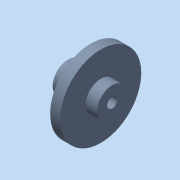
# Autodesk Inventor part: Kupplung
Saved by Autodesk Inventor 2015 (Build 190159000, 159)
## iProperties
Created: 2017-11-12
Part Number: Kupplung
Material: Generisch
Document SubType Name: Modeling
Designer: Christoph Soppa
Density: 1 g/cm^3
Appearance: Stahlblau - hell
Author: Christoph Soppa
Autodesk Inventor part; units mm, degrees
ref_plane "YZ Plane" through (0, 0, 0) normal (1, 0, 0) x (0, 1, 0)
ref_plane "XZ Plane" through (0, 0, 0) normal (0, 1, 0) x (-1, 0, 0)
ref_plane "XY Plane" through (0, 0, 0) normal (0, 0, 1) x (1, 0, 0)
sketch "Skizze1" plane through (0, 0, 0) normal (0, 0, 1) x (1, 0, 0)
  line L0 (0, 0) -> (16.2131, 0)
  line L1 (0, 2) -> (17.5, 2)
  line L2 (17.5, 2) -> (17.5, 6)
  line L3 (17.5, 6) -> (13, 6)
  line L4 (13, 6) -> (13, 16)
  line L5 (13, 16) -> (9, 16)
  line L6 (9, 16) -> (9, 6)
  line L7 (9, 6) -> (0, 6)
  line L8 (0, 6) -> (0, 2)
  dimension "d0" = 4
  dimension "d1" = 9
  dimension "d2" = 2
  dimension "d3" = 4.5
  dimension "d4" = 10
  dimension "d5" = 0
  dimension "d6" = 4
  dimension "d8" = 1.2869
  constraints: 18 end point, 6 perpendicular, 2 horizontal, 2 point on line
  measures "d0" distance of L7.end L1.start
  measures "d1" distance of L6.end L7.end
  measures "d2" distance between parallel lines of L1 L0
  measures "d3" distance of L2.end L3.end
  measures "d4" distance of L3.end L4.end
  measures "d5" distance from line of L8 L0.start
  measures "d6" distance of L4.end L5.end
  measures "d8" distance from line of L0.end L2
revolve "Umdrehung1" add sketch "Skizze1" angle 360 about axis through (0, 0, 0) along (1, 0, 0)
